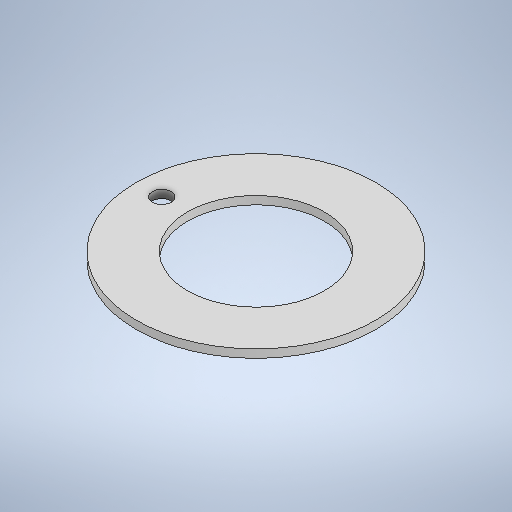
# Autodesk Inventor part: 42-02-005
Saved by Autodesk Inventor 2025.2 (Build 292293000, 293)
## iProperties
Created: 2024-11-14
Part Number: 42-02-005
Material: Generic
Document SubType Name: Modeling
Designer: Zvonko.Gabric
Density: 1 g/cm^3
Appearance: Default
Author: Zvonko.Gabric
Autodesk Inventor part; units mm, degrees
ref_plane "YZ Plane" through (0, 0, 0) normal (1, 0, 0) x (0, 1, 0)
ref_plane "XZ Plane" through (0, 0, 0) normal (0, 1, 0) x (-1, 0, 0)
ref_plane "XY Plane" through (0, 0, 0) normal (0, 0, 1) x (1, 0, 0)
sketch "Sketch2" plane through (0, 0, 0) normal (0, 1, 0) x (-1, 0, 0)
  circle A0 centre (0, 0) radius 22.2
  circle A1 centre (0, 0) radius 12.7
  circle A2 centre (17.5, 0) radius 1.75
  dimension "d40" = 44.4
  dimension "d41" = 25.4
  dimension "d42" = 3.5
  dimension "d43" = 17.5
  constraints: 3 centre point, 2 coincident
  measures "d40" diameter of A0
  measures "d41" diameter of A1
  measures "d42" diameter of A2
  measures "d43" distance of point (0, 0) A2.centre
extrude "Extrusion1" add sketch "Sketch2" along normal blind 1.5
body "Solid1"
